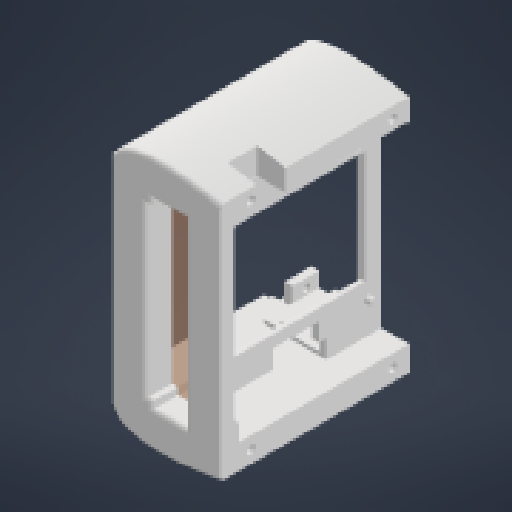
# Autodesk Inventor part: BP_BackHSCover
Saved by Autodesk Inventor 2026.1 (Build 301233020, 233B)
## iProperties
Created: 2025-09-12
Part Number: BP_BackHSCover
Material: Generic
Document SubType Name: Modeling
Designer: atrus
Density: 1 g/cm^3
Appearance: Default
Author: atrus
Autodesk Inventor part; units mm, degrees
ref_plane "YZ Plane" through (0, 0, 0) normal (1, 0, 0) x (0, 1, 0)
ref_plane "XZ Plane" through (0, 0, 0) normal (0, 1, 0) x (-1, 0, 0)
ref_plane "XY Plane" through (0, 0, 0) normal (0, 0, 1) x (1, 0, 0)
ref_plane "Work Plane1" through (0, 0, 0) normal (0, 0, 1) x (1, 0, 0)
sketch "Sketch1" plane through (0, 0, 0) normal (0, 0, 1) x (1, 0, 0)
  line L0 (-13.535, 44.65) -> (-5.515, 44.65) projected
  line L1 (-13.535, 37.45) -> (-13.535, 44.65) projected
  line L2 (-5.515, 44.65) -> (-5.515, 41.1825) projected
  line L3 (-5.515, 41.1825) -> (-2.515, 41.1825) projected
  line L4 (-2.515, 41.1825) -> (-2.515, 44.65) projected
  line L5 (-2.515, 44.65) -> (13.535, 44.65) projected
  line L6 (17.335, 46.4) -> (30.735, 46.4) projected
  line L7 (-13.535, -44.65) -> (-13.535, -37.45) projected
  line L8 (-5.515, -44.65) -> (-13.535, -44.65) projected
  line L9 (-2.515, -44.65) -> (-2.515, -41.1825) projected
  line L10 (-2.515, -41.1825) -> (-5.515, -41.1825) projected
  line L11 (-5.515, -41.1825) -> (-5.515, -44.65) projected
  line L12 (13.535, -44.65) -> (-2.515, -44.65) projected
  line L13 (30.735, -46.4) -> (17.335, -46.4) projected
  line L14 (17.135, 44.65) -> (17.135, 46.4)
  line L15 (17.135, 46.4) -> (17.335, 46.4)
  line L16 (17.335, 6.8007) -> (17.335, 46.4) construction
  line L17 (17.135, -44.65) -> (17.135, -46.4)
  line L18 (17.135, -46.4) -> (17.335, -46.4)
  line L19 (17.135, -44.65) -> (13.535, -44.65)
  line L20 (13.535, -44.65) -> (13.535, -22.65)
  line L21 (13.535, -22.65) -> (17.135, -22.65)
  line L22 (17.135, -22.65) -> (17.135, -44.65)
  line L23 (13.535, -22.65) -> (17.135, -22.65)
  line L24 (17.135, 44.65) -> (17.135, 32.65)
  line L25 (17.135, 32.65) -> (13.535, 32.65)
  line L26 (13.535, 32.65) -> (13.535, 44.65)
  spline S0 degree 3 poles (-23.335, 49.666) (-23.335, 50.975) (-23.1158, 52.2518) (-22.1621, 54.5446) (-21.5119, 55.5038) (-19.6866, 57.4002) (-18.4624, 58.2349) (-14.9112, 60.0651) (-12.2996, 60.7932) (-3.9024, 62.3581) (2.9614, 62.2896) (16.1612, 61.3119) (23.6495, 60.132) (30.735, 58.666) knots 0 0 0 0 0.392711 0.392711 0.745066 0.745066 1.182429 1.182429 1.943815 1.943815 3.746632 3.746632 5.901581 5.901581 5.901581 5.901581 projected
  line L27 (30.735, 46.4) -> (30.735, 58.666) projected
  spline S1 degree 3 poles (30.735, -58.666) (16.2749, -61.6577) (2.7493, -62.92) (-10.5484, -61.2397) (-14.2593, -60.4269) (-18.6937, -58.1029) (-20.0214, -57.1557) (-21.8009, -55.0954) (-22.3693, -54.1505) (-23.1581, -51.9961) (-23.335, -50.8419) (-23.335, -49.666) knots 0 0 0 0 4.429907 4.429907 5.935686 5.935686 6.645454 6.645454 7.140328 7.140328 7.660637 7.660637 7.660637 7.660637 projected
  line L28 (30.735, -46.4) -> (30.735, -58.666) projected
  line L29 (-23.335, -37.45) -> (-13.535, -37.45)
  line L30 (-23.335, 37.45) -> (-13.535, 37.45)
  line L31 (-23.335, 49.666) -> (-23.335, 37.45) projected
  line L32 (-23.335, -37.45) -> (-23.335, -49.666) projected
  point P0 (0, 0)
  dimension "d0" = 0.2
  dimension "d13" = 22
  dimension "d15" = 3.6
  dimension "d16" = 12
  constraints: 28 end point, 4 parallel, 4 perpendicular, 2 collinear, 1 horizontal
  measures "d0" distance between parallel lines of L16 L14
  measures "d13" distance of L19.end L20.end
  measures "d15" distance between parallel lines of L22 L20
  measures "d16" distance from line of L5.end L25
extrude "Main" add sketch "Sketch1" against normal blind 80
sketch "Sketch2" plane through (0, 0, 0) normal (0, 0, 1) x (1, 0, 0)
  line L0 (17.335, 47.5) -> (18.7552, 47.5) construction
  line L1 (18.7552, 44.5) -> (18.7552, 47.5) construction
  line L2 (17.335, 47.5) -> (17.335, 44.5) construction
  line L3 (30.735, 44.2166) -> (30.735, 47.7)
  line L4 (30.735, 47.7) -> (17.135, 47.7)
  line L5 (17.135, 47.7) -> (17.135, 44.2166)
  line L6 (17.135, 44.2166) -> (30.735, 44.2166)
  line L7 (17.135, 32.65) -> (17.135, 46.4) projected
  point P0 (0, 0)
  point P1 (17.135, 44.65)
  point P2 (30.735, 46.4)
  dimension "d3" = 0.2
  constraints: 8 end point, 3 perpendicular, 1 collinear, 1 point on line, 1 vertical
  measures "d3" distance between parallel lines of L4 L0
extrude "PCBCut" cut sketch "Sketch2" against normal blind 80
sketch "Sketch3" plane through (17.135, 47.7, 0) normal (0, -1, 0) x (1, 0, 0)
  line L0 (4.5548, -15.372) -> (4.5548, -8.992) construction
  arc A0 (4.5548, -8.992) -> (3.5748, -8.012) centre (3.5748, -8.992) ccw construction
  arc A1 (3.5748, -16.352) -> (4.5548, -15.372) centre (3.5748, -15.372) ccw construction
  line L1 (1.6202, -77) -> (1.6202, 2) construction
  line L2 (2.6202, -5.012) -> (13.6, -5.012)
  line L3 (13.6, -5.012) -> (13.6, -19.352)
  line L4 (13.6, -19.352) -> (2.6202, -19.352)
  line L5 (1.6202, -18.352) -> (1.6202, -6.012)
  line L6 (13.6, 0) -> (13.6, -80) construction
  line L7 (13.6, 0) -> (13.6, -80) projected
  line L8 (1.6202, -6.012) -> (1.6202, -5.012)
  line L9 (2.6202, -5.012) -> (1.6202, -5.012)
  line L10 (1.6202, -18.352) -> (1.6202, -19.352)
  line L11 (2.6202, -19.352) -> (1.6202, -19.352)
  point P0 (-17.135, 0)
  point P1 (13.6, -12.182)
  dimension "d6" = 3
  dimension "d7" = 3
  constraints: 18 end point, 5 point on line, 2 horizontal, 2 parallel, 2 perpendicular, 1 collinear, 1 midpoint
  measures "d6" distance from line of L2 A0.end
  measures "d7" distance from line of L4 A1.start
extrude "USBCCut" cut sketch "Sketch3" against normal blind 80
sketch "Sketch4" plane through (0, 0, 0) normal (0, 0, 1) x (1, 0, 0)
  line L0 (17.135, 47.7) -> (30.735, 47.7) projected
  line L1 (-23.335, 49.666) -> (-23.335, 37.45) projected
  line L2 (-23.335, 37.45) -> (-13.535, 37.45) projected
  line L3 (-13.535, 37.45) -> (-13.535, 44.65) projected
  line L4 (-13.535, 44.65) -> (-5.515, 44.65) projected
  line L5 (-5.515, 44.65) -> (-5.515, 41.1825) projected
  line L6 (-5.515, 41.1825) -> (-2.515, 41.1825) projected
  line L7 (-2.515, 41.1825) -> (-2.515, 44.65) projected
  line L8 (-2.515, 44.65) -> (13.535, 44.65) projected
  line L9 (17.135, 32.65) -> (17.135, 47.7) projected
  line L10 (17.135, -22.65) -> (13.535, -22.65) projected
  line L11 (13.535, -22.65) -> (13.535, -44.65) projected
  line L12 (13.535, 44.65) -> (13.535, 32.65) projected
  line L13 (13.535, 32.65) -> (17.135, 32.65) projected
  line L14 (30.735, 47.7) -> (30.735, 58.666) projected
  spline S0 degree 3 poles (30.735, 58.666) (23.6495, 60.132) (16.1612, 61.3119) (2.9614, 62.2896) (-3.9024, 62.3581) (-12.2996, 60.7932) (-14.9112, 60.0651) (-18.4624, 58.2349) (-19.6866, 57.4002) (-21.5119, 55.5038) (-22.1621, 54.5446) (-23.1158, 52.2518) (-23.335, 50.975) (-23.335, 49.666) knots 0 0 0 0 0.365148 0.365148 0.670628 0.670628 0.799642 0.799642 0.873752 0.873752 0.933457 0.933457 1 1 1 1 projected
  line L15 (13.535, -44.65) -> (-2.515, -44.65) projected
  line L16 (-2.515, -44.65) -> (-2.515, -41.1825) projected
  line L17 (-2.515, -41.1825) -> (-5.515, -41.1825) projected
  line L18 (-5.515, -41.1825) -> (-5.515, -44.65) projected
  line L19 (-5.515, -44.65) -> (-13.535, -44.65) projected
  line L20 (-13.535, -44.65) -> (-13.535, -37.45) projected
  line L21 (-13.535, -37.45) -> (-23.335, -37.45) projected
  line L22 (-23.335, -37.45) -> (-23.335, -49.666) projected
  spline S1 degree 3 poles (-23.335, -49.666) (-23.335, -50.8419) (-23.1581, -51.9961) (-22.3693, -54.1505) (-21.8009, -55.0954) (-20.0214, -57.1557) (-18.6937, -58.1029) (-14.2593, -60.4269) (-10.5484, -61.2397) (2.7493, -62.92) (16.2749, -61.6577) (30.735, -58.666) knots 0 0 0 0 0.06792 0.06792 0.132519 0.132519 0.225171 0.225171 0.421731 0.421731 1 1 1 1 projected
  line L23 (30.735, -58.666) -> (30.735, -46.4) projected
  line L24 (30.735, -46.4) -> (17.135, -46.4) projected
  line L25 (17.135, -46.4) -> (17.135, -22.65) projected
  point P0 (0, 0)
  constraints: 2 other
extrude "EndExt" add sketch "Sketch4" along normal blind 3.6
ref_plane "Work Plane2" through (0, 0, 0.2) normal (0, 0, 1) x (1, 0, 0)
sketch "Sketch7" plane through (0, 0, 3.6) normal (0, 0, 1) x (1, 0, 0)
  line L0 (-13.535, 37.45) -> (-13.535, 44.65)
  line L1 (-23.335, 37.45) -> (-13.535, 37.45)
  line L2 (-23.335, 46.4) -> (-23.335, 37.45)
  line L3 (-23.335, 46.4) -> (-1.335, 46.4)
  line L4 (-1.335, 46.4) -> (-1.335, 44.65)
  line L5 (-2.515, 44.65) -> (-1.335, 44.65)
  line L6 (-2.515, 41.1825) -> (-2.515, 44.65)
  line L7 (-5.515, 41.1825) -> (-2.515, 41.1825)
  line L8 (-5.515, 44.65) -> (-5.515, 41.1825)
  line L9 (-13.535, 44.65) -> (-5.515, 44.65)
  line L10 (30.735, 47.7) -> (30.735, 58.666) projected
  spline S0 degree 3 poles (30.735, 58.666) (23.6495, 60.132) (16.1612, 61.3119) (2.9614, 62.2896) (-3.9024, 62.3581) (-12.2996, 60.7932) (-14.9112, 60.0651) (-18.4624, 58.2349) (-19.6866, 57.4002) (-21.5119, 55.5038) (-22.1621, 54.5446) (-23.1158, 52.2518) (-23.335, 50.975) (-23.335, 49.666) knots 0 0 0 0 0.365148 0.365148 0.670628 0.670628 0.799642 0.799642 0.873752 0.873752 0.933457 0.933457 1 1 1 1 projected
  line L11 (-23.335, 49.666) -> (-23.335, 37.45) projected
  line L12 (-23.335, 37.45) -> (-13.535, 37.45) projected
  line L13 (-13.535, 37.45) -> (-13.535, 44.65) projected
  line L14 (-13.535, 44.65) -> (-5.515, 44.65) projected
  line L15 (-5.515, 44.65) -> (-5.515, 41.1825) projected
  line L16 (-5.515, 41.1825) -> (-2.515, 41.1825) projected
  line L17 (-2.515, 41.1825) -> (-2.515, 44.65) projected
  line L18 (-2.515, 44.65) -> (13.535, 44.65) projected
  line L19 (13.535, 44.65) -> (13.535, 32.65) projected
  line L20 (13.535, 32.65) -> (17.135, 32.65) projected
  line L21 (17.135, 32.65) -> (17.135, 47.7) projected
  line L22 (17.135, 47.7) -> (30.735, 47.7) projected
  line L23 (13.535, -22.65) -> (13.535, -44.65) projected
  line L24 (13.535, -44.65) -> (-2.515, -44.65) projected
  line L25 (-2.515, -44.65) -> (-2.515, -41.1825) projected
  line L26 (-2.515, -41.1825) -> (-5.515, -41.1825) projected
  line L27 (-5.515, -41.1825) -> (-5.515, -44.65) projected
  line L28 (-5.515, -44.65) -> (-13.535, -44.65) projected
  line L29 (-13.535, -44.65) -> (-13.535, -37.45) projected
  line L30 (-13.535, -37.45) -> (-23.335, -37.45) projected
  line L31 (-23.335, -37.45) -> (-23.335, -49.666) projected
  spline S1 degree 3 poles (-23.335, -49.666) (-23.335, -50.8419) (-23.1581, -51.9961) (-22.3693, -54.1505) (-21.8009, -55.0954) (-20.0214, -57.1557) (-18.6937, -58.1029) (-14.2593, -60.4269) (-10.5484, -61.2397) (2.7493, -62.92) (16.2749, -61.6577) (30.735, -58.666) knots 0 0 0 0 0.06792 0.06792 0.132519 0.132519 0.225171 0.225171 0.421731 0.421731 1 1 1 1 projected
  line L32 (30.735, -58.666) -> (30.735, -46.4) projected
  line L33 (30.735, -46.4) -> (17.135, -46.4) projected
  line L34 (17.135, -46.4) -> (17.135, -22.65) projected
  line L35 (17.135, -22.65) -> (13.535, -22.65) projected
  line L36 (-5.515, 41.1825) -> (-5.515, -41.1825)
  line L37 (-23.335, 37.45) -> (-23.335, -37.45)
  line L38 (13.535, 32.65) -> (13.535, -22.65)
  line L39 (30.735, 47.7) -> (30.735, -46.4)
  constraints: 28 end point, 2 parallel, 2 vertical, 2 other
extrude "Endcap" add sketch "Sketch7" along normal blind 9 contours L1 L2 L3 L4 L5 L6 L7 L8 L9 L0 | L0 L9 L8 L36 L27 L28 L29 L30 L37 L1 | L11 S0 L10 L22 L21 L20 L19 L18 L4 L3 | L30 L29 L28 L27 L26 L25 L24 L23 L35 L34 L33 L32 S1 L31 | L39 L33 L34 L35 L38 L20 L21 L22
fillet "Fillet1" radius 2 10 edges at (-23.335, 0, 12.6) (-2.9539, -62.0389, 12.6) (0.6695, 62.1456, 12.6) (13.535, 0, 12.6) (5.51, 44.65, 12.6) (-2.515, 42.9163, 12.6) (-4.015, 41.1825, 12.6) (-5.515, 0, 12.6) (-4.015, -41.1825, 12.6) (5.51, -44.65, 12.6)
sketch "Sketch8" plane through (17.135, -46.4, -80) normal (1, 0, 0) x (0, 0, -1)
  line L0 (0, 0) -> (-80.2, 0) projected
  line L1 (0, 8.95) -> (-80.2, 8.95) projected
  line L2 (-73.2, 0) -> (-27, 0)
  line L3 (-27, 0) -> (-27, 8.95)
  line L4 (-27, 8.95) -> (-73.2, 8.95)
  line L5 (-73.2, 8.95) -> (-73.2, 0)
  line L6 (-80.2, 0) -> (-80.2, 94.1) projected
  line L7 (0, 23.75) -> (0, 0) projected
  point P0 (-80, 46.4)
  point P1 (-27, 4.475)
  point P2 (-73.2, 8.95)
  dimension "d21" = 7
  dimension "d22" = 27
  constraints: 8 end point, 2 parallel, 2 point on line, 1 horizontal, 1 midpoint, 1 perpendicular
  measures "d21" distance between parallel lines of L6 L5
  measures "d22" distance from line of L7 point (-27, 4.475)
extrude "CutCord1" cut sketch "Sketch8" against normal blind 45 contours L0 L5 L1 L3
sketch "Sketch9" plane through (-23.335, -49.666, -80) normal (-1, 0, 0) x (0, 0, 1)
  line L0 (73.2, 87.116) -> (27, 87.116)
  line L1 (27, 87.116) -> (27, 96.066)
  line L2 (27, 96.066) -> (73.2, 96.066)
  line L3 (73.2, 96.066) -> (73.2, 87.116)
  line L4 (0, 87.116) -> (80.2, 87.116) projected
  line L5 (27, 3.266) -> (27, 12.216) projected
  line L6 (73.2, 12.216) -> (73.2, 3.266) projected
  point P0 (80, 49.666)
  point P1 (73.2, 91.591)
  dimension "d68" = 7
  constraints: 8 end point, 3 collinear, 2 parallel, 1 horizontal, 1 midpoint, 1 perpendicular
  measures "d68" horizontal distance of L4.end point (73.2, 91.591)
extrude "CutCord2" cut sketch "Sketch9" against normal blind 22
sketch "Sketch10" plane through (0, 0, 12.6) normal (0, 0, 1) x (1, 0, 0)
  line L0 (-5.515, 41.1825) -> (-2.515, 41.1825) projected
  line L1 (-6.815, -44.65) -> (-6.815, 44.65) projected
  line L2 (-2.515, 41.1825) -> (-6.815, 41.1825)
  line L3 (-6.815, 41.1825) -> (-6.815, 44.65)
  line L4 (-6.815, 44.65) -> (-2.515, 44.65)
  line L5 (-2.515, 44.65) -> (-2.515, 41.1825)
  line L6 (-2.515, -41.1825) -> (-5.515, -41.1825) projected
  line L7 (-5.515, -44.65) -> (-13.535, -44.65) projected
  line L8 (-2.515, -41.1825) -> (-6.815, -41.1825)
  line L9 (-6.815, -41.1825) -> (-6.815, -44.65)
  line L10 (-6.815, -44.65) -> (-2.515, -44.65)
  line L11 (-2.515, -44.65) -> (-2.515, -41.1825)
  point P0 (0, 0)
  constraints: 16 end point, 4 parallel, 2 horizontal, 2 perpendicular, 2 point on line
extrude "Extrusion8" add sketch "Sketch10" against normal up to surface (9 mm away)
fillet "Fillet2" radius 2 6 edges at (-2.515, 42.9163, 12.6) (-4.665, 41.1825, 12.6) (-4.665, -41.1825, 12.6) (-2.515, -43.9163, 12.6) (13.535, 32.65, -38.2) (13.535, -22.65, -38.2)
sketch "Sketch12" plane through (30.735, -48.4, 0.2) normal (1, 0, 0) x (0, 0, -1)
  circle A0 centre (4.24, 93.4) radius 0.508 projected
  circle A1 centre (1.7, 93.4) radius 0.508 projected
  circle A2 centre (73.45, 17.65) radius 1.8 projected
  circle A3 centre (1.95, 17.65) radius 1.8 projected
  circle A4 centre (73.45, 89.15) radius 1.8 projected
  circle A5 centre (1.95, 89.15) radius 1.8 projected
  circle A6 centre (15.272, 90.786) radius 0.325 projected
  circle A7 centre (9.492, 90.786) radius 0.325 projected
  arc A8 (7.762, 94.066) -> (8.362, 94.066) centre (8.062, 94.066) ccw projected
  line L0 (7.762, 94.066) -> (7.762, 94.866) projected
  arc A9 (8.362, 94.866) -> (7.762, 94.866) centre (8.062, 94.866) ccw projected
  line L1 (8.362, 94.866) -> (8.362, 94.066) projected
  arc A10 (16.402, 94.066) -> (17.002, 94.066) centre (16.702, 94.066) ccw projected
  line L2 (16.402, 94.066) -> (16.402, 94.866) projected
  arc A11 (17.002, 94.866) -> (16.402, 94.866) centre (16.702, 94.866) ccw projected
  line L3 (17.002, 94.866) -> (17.002, 94.066) projected
  arc A12 (7.762, 89.736) -> (8.362, 89.736) centre (8.062, 89.736) ccw projected
  line L4 (7.762, 89.736) -> (7.762, 90.836) projected
  arc A13 (8.362, 90.836) -> (7.762, 90.836) centre (8.062, 90.836) ccw projected
  line L5 (8.362, 90.836) -> (8.362, 89.736) projected
  arc A14 (16.402, 89.736) -> (17.002, 89.736) centre (16.702, 89.736) ccw projected
  line L6 (16.402, 89.736) -> (16.402, 90.836) projected
  arc A15 (17.002, 90.836) -> (16.402, 90.836) centre (16.702, 90.836) ccw projected
  line L7 (17.002, 90.836) -> (17.002, 89.736) projected
  circle A16 centre (44.2, 75.9) radius 0.625 projected
  circle A17 centre (46.74, 73.74) radius 0.51 projected
  circle A18 centre (44.2, 73.74) radius 0.51 projected
  circle A19 centre (41.66, 73.74) radius 0.51 projected
  circle A20 centre (39.12, 73.74) radius 0.51 projected
  circle A21 centre (67.002, 89.87) radius 0.51 projected
  circle A22 centre (67.002, 86.87) radius 0.51 projected
  circle A23 centre (64.002, 89.87) radius 0.51 projected
  circle A24 centre (64.002, 86.87) radius 0.51 projected
  circle A25 centre (63.062, 83.87) radius 0.51 projected
  circle A26 centre (63.062, 92.87) radius 0.51 projected
  line L8 (-1.8, 10.9) -> (77.2, 10.9) projected
  arc A27 (77.2, 10.9) -> (80.2, 13.9) centre (77.2, 13.9) ccw projected
  line L9 (80.2, 13.9) -> (80.2, 92.9) projected
  arc A28 (80.2, 92.9) -> (77.2, 95.9) centre (77.2, 92.9) ccw projected
  line L10 (77.2, 95.9) -> (-1.8, 95.9) projected
  arc A29 (-1.8, 95.9) -> (-4.8, 92.9) centre (-1.8, 92.9) ccw projected
  line L11 (-4.8, 92.9) -> (-4.8, 13.9) projected
  arc A30 (-4.8, 13.9) -> (-1.8, 10.9) centre (-1.8, 13.9) ccw projected
  line L12 (-1.8, 96.7) -> (77.2, 96.7)
  arc A31 (81, 92.9) -> (77.2, 96.7) centre (77.2, 92.9) ccw
  line L13 (81, 92.9) -> (81, 13.9)
  arc A32 (77.2, 10.1) -> (81, 13.9) centre (77.2, 13.9) ccw
  line L14 (77.2, 10.1) -> (-1.8, 10.1)
  arc A33 (-5.6, 13.9) -> (-1.8, 10.1) centre (-1.8, 13.9) ccw
  line L15 (-5.6, 13.9) -> (-5.6, 92.9)
  arc A34 (-1.8, 96.7) -> (-5.6, 92.9) centre (-1.8, 92.9) ccw
  dimension "d86" = 0.8
  constraints: 8 end point, 8 point on circle, 4 centre point, 7 other
  measures "d86" distance between parallel lines of L10 L12
extrude "EdgePCBCut" cut sketch "Sketch12" against normal up to surface (13.6 mm away) contours A0 | A1 | A2 | A3 | A4 | A5 | A6 | A7 | L0 A9 L1 A8 | L2 A11 L3 A10 | L4 A13 L5 A12 | L6 A15 L7 A14 | A16 | A17 | A18 | A19 | A20 | A21 | A22 | A23 | A24 | A25 | A26 | A30 L11 A29 L10 A28 L9 A27 L8 | L12 A31 L13 A32 L14 A33 L15 A34
sketch "Sketch13" plane through (17.135, -46.4, -80) normal (1, 0, 0) x (0, 0, -1)
  line L0 (-9, 93.9) -> (-20, 93.9)
  line L1 (-20, 93.9) -> (-20, 80.9)
  line L2 (-20, 80.9) -> (-9, 80.9)
  line L3 (-9, 80.9) -> (-9, 93.9)
  line L4 (0, 94.1) -> (0, 79.05) projected
  line L5 (-3, 93.9) -> (-82, 93.9) projected
  line L6 (-3, 93.9) -> (-82, 93.9) projected
  point P0 (-80, 46.4)
  point P1 (-14.5, 93.9)
  dimension "d39" = 13
  dimension "d40" = 9
  dimension "d41" = 11
  constraints: 8 end point, 2 parallel, 1 horizontal, 1 midpoint, 1 perpendicular, 1 point on line
  measures "d39" distance of L2.end L0.start
  measures "d40" distance between parallel lines of L4 L3
  measures "d41" distance of L1.end L2.end
extrude "PowerPinsCutout" cut sketch "Sketch13" against normal blind 10
sketch "Sketch11" plane through (17.135, -46.4, -80) normal (1, 0, 0) x (0, 0, -1)
  circle A0 centre (-6.75, 87.15) radius 1.8 construction
  circle A1 centre (-78.25, 87.15) radius 1.8 construction
  circle A2 centre (-78.25, 15.65) radius 1.8 construction
  circle A3 centre (-6.75, 15.65) radius 1.8 construction
  circle A4 centre (-6.75, 87.15) radius 1.7
  circle A5 centre (-6.75, 15.65) radius 1.7
  circle A6 centre (-78.25, 87.15) radius 1.7
  circle A7 centre (-78.25, 15.65) radius 1.7
  point P0 (-80, 46.4)
  dimension "d33" = 0.1
  constraints: 4 centre point, 4 coincident, 3 equal radius
  measures "d33" radial gap between concentric circles of A4 A0
extrude "PCBBoss" add sketch "Sketch11" along normal blind 3
sketch "Sketch14" plane through (0, 0, -80) normal (0, 0, -1) x (-1, 0, 0)
  arc A0 (-15.535, 32.65) -> (-13.535, 34.65) centre (-15.535, 34.65) ccw projected
  line L0 (-17.135, -22.65) -> (-17.135, -46.4) projected
  line L1 (-13.535, 34.65) -> (-17.135, 34.65)
  line L2 (-17.135, 34.65) -> (-17.135, -24.65)
  line L3 (-17.135, -24.65) -> (-13.535, -24.65)
  line L4 (-13.535, -24.65) -> (-13.535, 34.65)
  point P0 (0, 0)
  constraints: 8 end point, 2 parallel, 1 horizontal, 1 perpendicular, 1 point on circle, 1 point on line
extrude "Extrusion12" add sketch "Sketch14" against normal blind 8
fillet "Fillet4" radius 2 3 edges at (13.535, 39.6499, -80) (13.535, 5, -80) (13.535, -34.6499, -80)
sketch "Sketch15" plane through (-23.335, -49.666, -80) normal (-1, 0, 0) x (0, 0, 1)
  line L0 (0, 12.216) -> (80.2, 12.216) projected
  line L1 (0, 0) -> (85.5, 0) projected
  line L2 (0, 12.216) -> (13, 12.216)
  line L3 (13, 12.216) -> (13, 0)
  line L4 (13, 0) -> (0, 0)
  line L5 (0, 0) -> (0, 12.216)
  line L6 (83.6, 87.116) -> (0, 87.116) projected
  line L7 (0, 99.332) -> (90.6, 99.332) projected
  line L8 (0, 87.116) -> (13, 87.116)
  line L9 (13, 87.116) -> (13, 99.332)
  line L10 (13, 99.332) -> (0, 99.332)
  line L11 (0, 99.332) -> (0, 87.116)
  point P0 (80, 49.666)
  point P1 (27, 12.216)
  point P2 (27, 87.116)
  point P3 (85.5, 99.332)
  point P4 (0, 6.108)
  point P5 (13, 87.116)
  point P6 (13, 12.216)
  point P7 (94.5, 99.332)
  point P8 (84.5, 87.116)
  dimension "d48" = 13
  constraints: 16 end point, 4 parallel, 2 horizontal, 2 perpendicular, 2 point on line, 1 collinear, 1 midpoint
  measures "d48" distance from line of point (0, 6.108) L3
extrude "Extrusion13" cut sketch "Sketch15" against normal blind 6
sketch "Sketch16" plane through (-17.335, -49.666, -80) normal (-1, 0, 0) x (0, 0, 1)
  line L0 (13, 0) -> (0, 0) construction
  line L1 (13, 99.332) -> (90.6, 99.332) construction
  line L2 (0, 12.216) -> (13, 12.216) projected
  line L3 (13, 87.116) -> (0, 87.116) projected
  line L4 (0, 87.116) -> (0, 99.332) projected
  point P0 (80, 49.666)
  point P1 (6, 91.616)
  point P2 (6, 7.716)
  point P3 (85.5, 99.332)
  point P4 (94.5, 99.332)
  dimension "d51" = 4.5
  dimension "d52" = 4.5
  dimension "d100" = 6
  constraints: 1 vertical alignment
  measures "d51" distance from line of L2 point (6, 7.716)
  measures "d52" distance from line of L3 point (6, 91.616)
  measures "d100" distance from line of L4 point (6, 91.616)
hole "Hole1" at (-17.335, 41.95, -74) at (-17.335, -41.95, -74) direction (1, 0, 0) diameter 3.6 depth 8 tip angle 118 clearance for "Flat Head Machine Screw" size "M3" standard "Ansi Metric M Profile"
sketch "Sketch17" plane through (0, 0, -80) normal (0, 0, -1) x (-1, 0, 0)
  line L0 (17.335, 45.65) -> (17.335, 49.666) projected
  line L1 (13.335, 45.65) -> (17.335, 45.65) projected
  line L2 (13.335, 48.65) -> (13.335, 45.65) projected
  line L3 (-29.735, 48.65) -> (13.335, 48.65) projected
  line L4 (-29.735, 52.65) -> (-29.735, 48.65) projected
  line L5 (17.335, 52.65) -> (-29.735, 52.65) projected
  line L6 (17.335, 49.666) -> (17.335, 52.65) projected
  line L7 (17.335, -45.65) -> (13.335, -45.65) projected
  line L8 (17.335, -49.666) -> (17.335, -45.65) projected
  line L9 (17.335, -52.65) -> (17.335, -49.666) projected
  line L10 (-29.735, -52.65) -> (17.335, -52.65) projected
  line L11 (-29.735, -48.65) -> (-29.735, -52.65) projected
  line L12 (13.335, -48.65) -> (-29.735, -48.65) projected
  line L13 (13.335, -45.65) -> (13.335, -48.65) projected
  point P0 (0, 0)
extrude "Extrusion14" cut sketch "Sketch17" against normal blind 2
sketch "Sketch18" plane through (30.735, -58.666, -80) normal (1, 0, 0) x (0, 0, -1)
  line L0 (0, 10.266) -> (-83.6, 10.266) construction
  line L1 (0, 0) -> (-85.5, 0) construction
  line L2 (0, 12.266) -> (0, 0) construction
  line L3 (0, 6.133) -> (-85.5, 6.133) construction
  line L4 (-60.648, 117.332) -> (0, 117.332) construction
  line L5 (-60.648, 106.366) -> (0, 106.366) construction
  line L6 (0, 117.332) -> (0, 106.366) construction
  line L7 (0, 111.849) -> (-85.5, 111.849) construction
  circle A0 centre (-8, 6.133) radius 2
  circle A1 centre (-77.5, 6.133) radius 2
  circle A2 centre (-8, 111.849) radius 2
  circle A3 centre (-77.5, 111.849) radius 2
  line L8 (-85.5, 0) -> (-85.5, 9) projected
  point P0 (-80, 58.666)
  point P1 (-83.6, 12.266)
  dimension "d62" = 8
  dimension "d63" = 8
  dimension "d64" = 4
  constraints: 5 point on line, 4 centre point, 4 end point, 3 equal radius, 2 horizontal, 2 midpoint, 2 vertical alignment
  measures "d62" distance from line of L2 A0.centre
  measures "d63" distance of L3.end A1.centre
  measures "d64" diameter of A0
extrude "Extrusion15" cut sketch "Sketch18" against normal blind 7
sketch "Sketch23" plane through (0, 0, 3.6) normal (0, 0, -1) x (-1, 0, 0)
  line L0 (23.335, 37.45) -> (13.535, 37.45)
  line L1 (13.535, 37.45) -> (13.535, -37.45)
  line L2 (13.535, -37.45) -> (23.335, -37.45)
  line L3 (23.335, -37.45) -> (23.335, 37.45)
  point P0 (0, 0)
  constraints: 8 end point, 2 parallel, 1 horizontal, 1 perpendicular
extrude "Extrusion20" add sketch "Sketch23" along normal blind 3.4
sketch "Sketch20" plane through (-23.335, -37.45, 3.6) normal (-1, 0, 0) x (0, 0, 1)
  line L0 (-70.6, 87.116) -> (-70.6, 74.9) construction
  line L1 (-56.6, 74.9) -> (-70.6, 74.9) construction
  line L2 (-56.6, 74.9) -> (-56.6, 83.85) construction
  line L3 (-56.6, 83.85) -> (-10.4, 83.85) construction
  line L4 (-10.4, 83.85) -> (-10.4, 74.9) construction
  line L5 (-3.4, 74.9) -> (-10.4, 74.9) construction
  line L6 (-70.6, 87.116) -> (7, 87.116) construction
  line L7 (-77.5763, -12.216) -> (7, -12.216)
  line L8 (-77.5763, -12.216) -> (7, -12.216) projected
  line L9 (7, 87.116) -> (-70.6, 87.116)
  line L10 (-70.6, 87.116) -> (-70.6, 85.316)
  line L11 (1.8, 85.316) -> (1.8, -10.416)
  line L12 (1.8, -10.416) -> (-77.5763, -10.416)
  line L13 (-77.5763, -12.216) -> (-77.5763, -10.416)
  line L14 (-70.6, 85.316) -> (1.8, 85.316)
  line L15 (-10.4, 0) -> (-3.4, 0) projected
  line L16 (-10.4, 0) -> (-10.4, -8.95) projected
  line L17 (-10.4, -8.95) -> (-56.6, -8.95) projected
  line L18 (-56.6, -8.95) -> (-56.6, 0) projected
  line L19 (-70.6, 0) -> (-56.6, 0) projected
  line L20 (-70.6, 0) -> (-70.6, -12.216) projected
  line L21 (-70.6, -12.216) -> (7, -12.216) projected
  line L22 (7, 87.116) -> (7, -12.216) projected
  line L23 (3.6, 87.116) -> (3.6, -12.216)
  line L24 (-3.4, 0) -> (-3.4, 74.9) projected
  point P0 (-3.6, 37.45)
  point P1 (-70.6, -10.416)
  dimension "d74" = 1.8
  dimension "d76" = 1.8
  dimension "d87" = 1.8
  dimension "d88" = 3.4
  constraints: 16 end point, 3 perpendicular, 3 point on line, 1 collinear
  measures "d74" distance between parallel lines of L6 L14
  measures "d76" distance between parallel lines of L7 L12
  measures "d87" distance between parallel lines of L11 L23
  measures "d88" distance between parallel lines of L22 L23
extrude "Extrusion17" add sketch "Sketch20" along normal blind 4 contours L20 L12 L11 L14 L10 L9 L23 L7
sketch "Sketch21" plane through (-23.335, -37.45, 3.6) normal (-1, 0, 0) x (0, 0, 1)
  circle A0 centre (-6.9, -3.5) radius 1.9
  circle A1 centre (-6.9, 78.4) radius 1.9
  circle A2 centre (-6.9, 78.4) radius 1.2295 projected
  circle A3 centre (-6.9, -3.5) radius 1.2295 projected
  point P0 (-3.6, 37.45)
  dimension "d79" = 3.8
  dimension "d80" = 3.8
  constraints: 2 centre point, 2 coincident
  measures "d79" diameter of A1
  measures "d80" diameter of A0
extrude "Extrusion18" cut sketch "Sketch21" against normal blind 10 contours A0 | A1 | A2 | A3
sketch "Sketch22" plane through (18.7552, 47.7, -6.012) normal (1, 0, 0) x (0, 0, -1)
  line L0 (-1, 0.6) -> (13.34, 0.6) projected
  line L1 (13.34, 0.6) -> (13.34, 13.0709) projected
  spline S0 degree 6 poles (-1, 13.0709) (-0.8333, 13.0709) (-0.6667, 13.0709) (-0.5, 13.0709) (-0.3333, 13.0709) (-0.1667, 13.0709) (1.5913, 13.0709) (3.7535, 13.0709) (6.2609, 13.0709) (8.8747, 13.0709) (11.1664, 13.0709) (12.5067, 13.0709) (12.6733, 13.0709) (12.84, 13.0709) (13.0067, 13.0709) (13.1733, 13.0709) (13.34, 13.0709) knots 0 0 0 0 0 0 0 0.084008 0.084008 0.084008 0.084008 0.084008 0.886091 0.886091 0.886091 0.886091 0.886091 1 1 1 1 1 1 1 projected
  line L2 (-1, 0.6) -> (-1, 13.0709) projected
  line L3 (13.34, 13.0709) -> (-1, 13.0709)
  line L4 (-1, 13.0709) -> (-1, 35.6972)
  line L5 (-1, 35.6972) -> (13.34, 35.6972)
  line L6 (13.34, 35.6972) -> (13.34, 13.0709)
  point P0 (-6.012, -47.7)
  constraints: 8 end point, 2 parallel, 1 horizontal, 1 perpendicular, 1 other
extrude "Extrusion19" cut sketch "Sketch22" against normal blind 2
sketch "Sketch24" plane through (13.535, -44.65, 10.6) normal (-1, 0, 0) x (0, 0, 1)
  line L0 (-39.225, 8.6) -> (-39.225, 14.2) projected
  line L1 (-57.975, 14.2) -> (-57.975, 8.6) projected
  line L2 (-59.975, 16.2) -> (-37.225, 16.2)
  line L3 (-37.225, 16.2) -> (-37.225, 5.6)
  line L4 (-37.225, 5.6) -> (-59.975, 5.6)
  line L5 (-59.975, 5.6) -> (-59.975, 16.2)
  point P0 (-10.6, 44.65)
  dimension "d91" = 2
  dimension "d92" = 2
  dimension "d93" = 2
  dimension "d94" = 3
  constraints: 8 end point, 2 parallel, 1 horizontal, 1 perpendicular
  measures "d91" distance between parallel lines of L5 L1
  measures "d92" distance between parallel lines of L3 L0
  measures "d93" distance from line of L2 L0.end
  measures "d94" distance from line of L0.start L4
extrude "Extrusion21" cut sketch "Sketch24" against normal blind 10
sketch "Sketch25" plane through (0, 0, 3.6) normal (0, 0, -1) x (-1, 0, 0)
  line L0 (13.535, -44.65) -> (13.535, 44.65) projected
  line L1 (13.535, 44.65) -> (5.515, 44.65) projected
  line L2 (5.515, 44.65) -> (5.515, 41.1825) projected
  line L3 (5.515, -41.1825) -> (5.515, 41.1825) projected
  line L4 (5.515, -41.1825) -> (5.515, -44.65) projected
  line L5 (5.515, -44.65) -> (13.535, -44.65) projected
  point P0 (0, 0)
extrude "Extrusion22" add sketch "Sketch25" along normal blind 3.4
fillet "Fillet7" radius 2 1 edges at (13.535, 5, 3.6)
sketch "Sketch26" plane through (-23.335, 37.45, -53) normal (0, -1, 0) x (1, 0, 0)
  line L0 (0, -14) -> (6, -14) projected
  line L1 (9.8, -27) -> (9.8, 0) projected
  line L2 (0, -14) -> (9.8, -14)
  line L3 (9.8, -14) -> (9.8, 0)
  line L4 (9.8, 0) -> (0, 0)
  line L5 (0, 0) -> (0, -14)
  point P0 (23.335, 53)
  constraints: 8 end point, 2 parallel, 1 horizontal, 1 perpendicular
extrude "Extrusion23" cut sketch "Sketch26" against normal up to surface (8.95 mm away)
sketch "Sketch27" plane through (-23.335, -37.45, -53) normal (0, 1, 0) x (1, 0, 0)
  line L0 (0, 14) -> (0, 0) projected
  line L1 (9.8, 27) -> (9.8, 0) projected
  line L2 (0, 14) -> (9.8, 14)
  line L3 (9.8, 14) -> (9.8, 0)
  line L4 (9.8, 0) -> (0, 0)
  line L5 (0, 0) -> (0, 14)
  point P0 (23.335, -53)
  constraints: 8 end point, 2 parallel, 1 horizontal, 1 perpendicular
extrude "Extrusion24" cut sketch "Sketch27" against normal up to surface (8.95 mm away)
body "Solid1"
